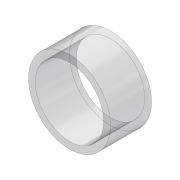
# Autodesk Inventor part: middleFlange
Saved by Autodesk Inventor 2018 (Build 220112000, 112)
## iProperties
Created: 2020-03-26
Part Number: middleFlange
Material: Polycarbonate, Clear
Document SubType Name: Modeling
Designer: Matt
Density: 1.2 g/cm^3
Appearance: Polycarbonate - Clear
Author: Matt
Autodesk Inventor part; units mm, degrees
ref_plane "YZ Plane" through (0, 0, 0) normal (1, 0, 0) x (0, 1, 0)
ref_plane "XZ Plane" through (0, 0, 0) normal (0, 1, 0) x (-1, 0, 0)
ref_plane "XY Plane" through (0, 0, 0) normal (0, 0, 1) x (1, 0, 0)
sketch "Sketch1" plane through (0, 0, 0) normal (0, 0, 1) x (1, 0, 0)
  circle A0 centre (0, 0) radius 15.875 projected
  circle A1 centre (0, 0) radius 19.05
  point P0 (0, 0)
  dimension "d0" = 38.1
  constraints: 1 centre point, 1 coincident
  measures "d0" diameter of A1
extrude "Extrusion1" add sketch "Sketch1" along normal blind 19.05
body "Solid1"
